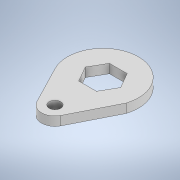
# Autodesk Inventor part: SP8V1 Conductor Hexagonal Freno
Saved by Autodesk Inventor 2021.2 (Build 252289000, 289)
## iProperties
Created: 2026-06-16
Part Number: SP8V1 Conductor Hexagonal Freno
Material: Generic
Document SubType Name: Sheet Metal
Designer: nelso
Density: 1 g/cm^3
Sheet Metal Rule: Default_mm
Appearance: Default
Author: nelso
Autodesk Inventor part; units mm, degrees
ref_plane "YZ Plane" through (0, 0, 0) normal (1, 0, 0) x (0, 1, 0)
ref_plane "XZ Plane" through (0, 0, 0) normal (0, 1, 0) x (-1, 0, 0)
ref_plane "XY Plane" through (0, 0, 0) normal (0, 0, 1) x (1, 0, 0)
sketch "Sketch1" plane through (0, 0, 0) normal (0, 1, 0) x (-1, 0, 0)
  circle A0 centre (0, 0) radius 3
  circle A1 centre (0, 0) radius 7
  circle A2 centre (0, -25) radius 18.5
  line L0 (6.2154, 3.22) -> (16.4265, -16.49)
  line L1 (-17.6376, -19.4175) -> (-6.2496, 3.1532)
  line L2 (9.2376, -25) -> (4.6188, -33)
  line L3 (4.6188, -33) -> (-4.6188, -33)
  line L4 (-4.6188, -33) -> (-9.2376, -25)
  line L5 (-9.2376, -25) -> (-4.6188, -17)
  line L6 (-4.6188, -17) -> (4.6188, -17)
  line L7 (4.6188, -17) -> (9.2376, -25)
  point P0 (4.4139, 5.433)
  point P1 (-13.2255, -12.0641)
  dimension "d3" = 6
  dimension "d6" = 14
  dimension "d11" = 25
  dimension "d12" = 37
  dimension "d13" = 16
  measures "d3" diameter of A0
  measures "d6" diameter of A1
  measures "d11" distance of A2.centre A0.centre
  measures "d12" diameter of A2
  measures "d13" distance between parallel lines of L3 L6
extrude "Plate1" add sketch "Sketch1" along normal mid plane 4.7 contours A1 A2 | A1 L0 A2 | A2 L1 A1 | A1 A2 | A1 A2 L1
equation "\"d9\" = Thickness"
equation "\"BendRadius\" = Thickness"
equation "\"BendReliefWidth\" = Thickness"
equation "\"BendReliefDepth\" = 0.5 * Thickness"
equation "\"CornerReliefSize\" = 4 * Thickness"
equation "\"MinimumRemnant\" = 2 * Thickness"
equation "\"TransitionRadius\" = BendRadius"
equation "\"JacobiRadiusSize\" = BendRadius"
equation "\"GapSize\" = Thickness"
equation "\"Thickness\" = 4.7"
body "Solid1"
